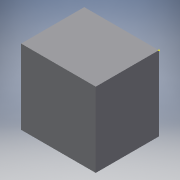
# Autodesk Inventor part: Power Cube
Saved by Autodesk Inventor 2018 (Build 220112000, 112)
## iProperties
Created: 2018-02-01
Part Number: Power Cube
Material: Generic
Document SubType Name: Modeling
Designer: Luke
Density: 1 g/cm^3
Appearance: Default
Author: Luke
Autodesk Inventor part; units mm, degrees
ref_plane "YZ Plane" through (0, 0, 0) normal (1, 0, 0) x (0, 1, 0)
ref_plane "XZ Plane" through (0, 0, 0) normal (0, 1, 0) x (-1, 0, 0)
ref_plane "XY Plane" through (0, 0, 0) normal (0, 0, 1) x (1, 0, 0)
sketch "Sketch1" plane through (0, 0, 0) normal (0, 0, 1) x (1, 0, 0)
  line L0 (0, 0) -> (-330.2, 0)
  line L1 (-330.2, 0) -> (-330.2, -330.2)
  line L2 (-330.2, -330.2) -> (0, -330.2)
  line L3 (0, -330.2) -> (0, 0)
  dimension "d0" = 330.2
  dimension "d1" = 330.2
  constraints: 8 end point, 2 parallel, 1 horizontal, 1 perpendicular
  measures "d0" distance of L2.end L1.end
  measures "d1" distance of L1.end L0.end
extrude "Extrusion1" add sketch "Sketch1" along normal blind 279.4
sketch "Sketch2" plane through (0, 0, 0) normal (0, 0, -1) x (-1, 0, 0)
  line L0 (22.1452, -202.8313) -> (121.2225, -202.8313) construction
  line L1 (121.2225, -202.8313) -> (121.2225, -254.2067) construction
  line L2 (121.2225, -254.2067) -> (22.1452, -254.2067) construction
  line L3 (22.1452, -254.2067) -> (22.1452, -202.8313) construction
  point P0 (0, 0)
  constraints: 2 other
body "Solid1"
